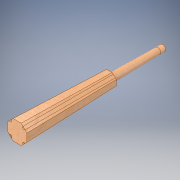
# Autodesk Inventor part: itomaki
Saved by Autodesk Inventor 2019 (Build 230136000, 136)
## iProperties
Created: 2019-11-15
Part Number: itomaki
Material: Клен
Document SubType Name: Modeling
Designer: stepa
Density: 0.705 g/cm^3
Appearance: Клен — массив — натуральный — с умеренным глянцем
Author: stepa
Autodesk Inventor part; units mm, degrees
ref_plane "YZ Plane" through (0, 0, 0) normal (1, 0, 0) x (0, 1, 0)
ref_plane "XZ Plane" through (0, 0, 0) normal (0, 1, 0) x (-1, 0, 0)
ref_plane "XY Plane" through (0, 0, 0) normal (0, 0, 1) x (1, 0, 0)
sketch "Эскиз1" plane through (0, 0, 0) normal (0, 0, 1) x (1, 0, 0)
  circle A0 centre (0, 0) radius 3
  dimension "d0" = 6
  constraints: 1 centre point, 1 coincident
  measures "d0" diameter of A0
extrude "Выдавливание1" add sketch "Эскиз1" along normal blind 5
sketch "Эскиз2" plane through (0, 0, 5) normal (0, 0, 1) x (1, 0, 0)
  circle A0 centre (0, 0) radius 4
  dimension "d3" = 8
  constraints: 1 centre point, 1 coincident
  measures "d3" diameter of A0
extrude "Выдавливание2" add sketch "Эскиз2" along normal blind 50
sketch "Эскиз3" plane through (0, 0, 55) normal (0, 0, 1) x (1, 0, 0)
  line L0 (-10, 4.142136) -> (-4.142136, 10)
  line L1 (-4.142136, 10) -> (4.142136, 10)
  line L2 (4.142136, 10) -> (10, 4.142136)
  line L3 (10, 4.142136) -> (10, -4.142136)
  line L4 (10, -4.142136) -> (4.142136, -10)
  line L5 (4.142136, -10) -> (-4.142136, -10)
  line L6 (-4.142136, -10) -> (-10, -4.142136)
  line L7 (-10, -4.142136) -> (-10, 4.142136)
  point P0 (0, 0)
  point P1 (0, 0)
  dimension "d6" = 20
  constraints: 16 end point, 1 coincident, 1 horizontal, 17 other
  measures "d6" distance between parallel lines of L3 L7
extrude "Выдавливание3" add sketch "Эскиз3" along normal blind 95
chamfer "Фаска1" distance 1 distance2 50 1 edges at (-4, 0, 5) measured on face at (-3.5, 0, 5)
chamfer "Фаска2" distance 3 angle 88.1912 8 edges at (7.0711, 7.0711, 55) (0, 10, 55) (-7.0711, 7.0711, 55) (-10, 0, 55) (-7.0711, -7.0711, 55) (0, -10, 55) (7.0711, -7.0711, 55) (10, 0, 55) measured on face at (-6.7175, -6.7175, 55) measured on face at (6.7175, 6.7175, 55) measured on face at (0, -9.5, 55) measured on face at (6.7175, -6.7175, 55) measured on face at (-6.7175, 6.7175, 55) measured on face at (9.5, 0, 55) measured on face at (0, 9.5, 55) measured on face at (-9.5, 0, 55)
ref_plane "РабПлоскость1" through (-7.071068, 7.071068, 150) normal (-0.0223186, 0.0223186, 0.9995018) x (-0.7071068, -0.7071068, 0)
sketch "Эскиз4" plane through (-7.071068, 7.071068, 150) normal (-0.0223186, 0.0223186, 0.9995018) x (-0.7071068, -0.7071068, 0)
  line L0 (-4.142136, 0) -> (4.142136, 0)
  arc A0 (1.5, 0) -> (-1.5, 0) centre (0, 0) ccw
  point P0 (0, 5.260536)
  dimension "d15" = 1.5
  constraints: 2 point on circle, 2 point on line, 1 centre point, 1 midpoint
  measures "d15" radius of A0
extrude "Выдавливание4" cut sketch "Эскиз4" against normal up to next
ref_plane "РабПлоскость2" through (7.071068, 7.071068, 150) normal (0.0223186, 0.0223186, 0.9995018) x (-0.7071068, 0.7071068, 0)
sketch "Эскиз5" plane through (7.071068, 7.071068, 150) normal (0.0223186, 0.0223186, 0.9995018) x (-0.7071068, 0.7071068, 0)
  line L0 (-4.142136, 0) -> (4.142136, 0)
  line L1 (-2.899495, 0) -> (2.899495, 0)
  arc A0 (1.5, 0) -> (-1.5, 0) centre (0, 0) ccw
  line L2 (1.5, 0) -> (-1.5, 0)
  point P0 (0, 5.260536)
  dimension "d18" = 1.5
  constraints: 2 end point, 2 point on circle, 1 centre point, 1 collinear, 1 midpoint, 1 point on line
  measures "d18" radius of A0
extrude "Выдавливание5" cut sketch "Эскиз5" against normal up to next
ref_plane "РабПлоскость3" through (7.071068, -7.071068, 150) normal (0.0223186, -0.0223186, 0.9995018) x (0.7071068, 0.7071068, 0)
ref_plane "РабПлоскость4" through (-7.071068, -7.071068, 150) normal (-0.0223186, -0.0223186, 0.9995018) x (0.7071068, -0.7071068, 0)
sketch "Эскиз6" plane through (7.071068, -7.071068, 150) normal (0.0223186, -0.0223186, 0.9995018) x (0.7071068, 0.7071068, 0)
  line L0 (-4.142136, 0) -> (4.142136, 0)
  arc A0 (1.5, 0) -> (-1.5, 0) centre (0, 0) ccw
  line L1 (1.5, 0) -> (-1.5, 0)
  point P0 (0, 5.260536)
  dimension "d21" = 1.5
  constraints: 2 end point, 2 point on circle, 2 point on line, 1 centre point, 1 collinear, 1 midpoint
  measures "d21" radius of A0
extrude "Выдавливание6" cut sketch "Эскиз6" against normal up to next
sketch "Эскиз7" plane through (-7.071068, -7.071068, 150) normal (-0.0223186, -0.0223186, 0.9995018) x (0.7071068, -0.7071068, 0)
  line L0 (-4.142136, 0) -> (4.142136, 0)
  arc A0 (1.5, 0) -> (-1.5, 0) centre (0, 0) ccw
  line L1 (-1.5, 0) -> (1.5, 0)
  point P0 (0, 5.260536)
  dimension "d24" = 1.5
  constraints: 2 end point, 2 point on circle, 2 point on line, 1 centre point, 1 horizontal, 1 midpoint
  measures "d24" radius of A0
extrude "Выдавливание7" cut sketch "Эскиз7" against normal up to next
